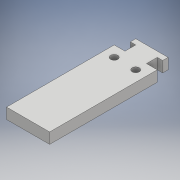
# Autodesk Inventor part: Attachment
Saved by Autodesk Inventor 2018 (Build 220112000, 112)
## iProperties
Created: 2018-05-09
Part Number: Attachment
Material: Generic
Document SubType Name: Modeling
Designer: s4321966
Density: 1 g/cm^3
Appearance: Default
Mass: 5.35187 g
Surface Area: 30.6948 cm^2
Volume: 5.35187 cm^3
Author: s4321966
Autodesk Inventor part; units mm, degrees
ref_plane "YZ Plane" through (0, 0, 0) normal (1, 0, 0) x (0, 1, 0)
ref_plane "XZ Plane" through (0, 0, 0) normal (0, 1, 0) x (-1, 0, 0)
ref_plane "XY Plane" through (0, 0, 0) normal (0, 0, 1) x (1, 0, 0)
sketch "Sketch1" plane through (0, 0, 0) normal (0, 0, 1) x (1, 0, 0)
  line L0 (0, 0) -> (20, 0)
  line L1 (20, 0) -> (20, -2.7984)
  line L2 (0, -2.7984) -> (0, 0)
  line L3 (0, 0) -> (20, 0)
  line L4 (20, 0) -> (20, -50)
  line L5 (20, -50) -> (0, -50)
  line L6 (0, -50) -> (0, 0)
  line L7 (0, 0) -> (5, 0)
  line L8 (0, -5) -> (0, 0)
  circle A0 centre (5, -5) radius 1.651
  line L9 (20, 0) -> (15, 0)
  line L10 (15, -5) -> (20, -5)
  line L11 (20, -5) -> (20, 0)
  circle A1 centre (15, -5) radius 1.651
  dimension "d1" = 20
  dimension "d2" = 50
  dimension "d6" = 5
  dimension "d7" = 5
  dimension "d9" = 3.302
  constraints: 24 end point, 4 horizontal, 4 parallel, 2 centre point, 2 perpendicular
  measures "d1" distance of L4.end L5.end
  measures "d2" distance of L3.end L4.end
  measures "d6" distance of L10.end L10.start
  measures "d7" distance of L10.start L9.end
  measures "d9" diameter of A1
extrude "Extrusion1" add sketch "Sketch1" along normal blind 5
sketch "Sketch2" plane through (0, 0, 5) normal (0, 0, 1) x (1, 0, 0)
  line L0 (20, 0) -> (0, 0) projected
  line L1 (10, 0) -> (5, 0)
  line L2 (5, 0) -> (5, 5)
  line L3 (5, 5) -> (10, 5)
  line L4 (10, 5) -> (10, 0)
  line L5 (10, 5) -> (2.5, 5)
  line L6 (2.5, 5) -> (2.5, 7.5)
  line L7 (2.5, 7.5) -> (10, 7.5)
  line L8 (10, 7.5) -> (10, 5)
  line L9 (2.5, 7.5) -> (17.5, 7.5)
  line L10 (17.5, 7.5) -> (17.5, 5)
  line L11 (17.5, 5) -> (2.5, 5)
  line L12 (2.5, 5) -> (2.5, 7.5)
  line L13 (10, 5) -> (15, 5)
  line L14 (15, 5) -> (15, 0)
  line L15 (15, 0) -> (10, 0)
  line L16 (10, 0) -> (10, 5)
  dimension "d12" = 5
  dimension "d13" = 5
  dimension "d14" = 7.5
  dimension "d15" = 2.5
  dimension "d16" = 15
  dimension "d17" = 2.5
  dimension "d18" = 5
  dimension "d19" = 5
  constraints: 32 end point, 8 parallel, 4 horizontal, 4 perpendicular, 1 midpoint
  measures "d12" distance of L2.end L3.end
  measures "d13" distance of L1.end L2.end
  measures "d14" distance of L6.end L7.end
  measures "d15" distance of L5.end L6.end
  measures "d16" distance of L10.end L11.end
  measures "d17" distance of L9.end L10.end
  measures "d18" distance of L14.end L15.end
  measures "d19" distance of L13.end L14.end
extrude "Extrusion2" add sketch "Sketch2" against normal blind 5
body "Solid1"
